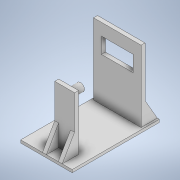
# Autodesk Inventor part: Część2
Saved by Autodesk Inventor 2022.2 (Build 262287010, 287A)
## iProperties
Created: 2023-01-23
Part Number: Część2
Material: Ogólny
Document SubType Name: Modeling
Designer: Miki
Density: 1 g/cm^3
Appearance: Domyślna
Author: Miki
Autodesk Inventor part; units mm, degrees
ref_plane "YZ Plane" through (0, 0, 0) normal (1, 0, 0) x (0, 1, 0)
ref_plane "XZ Plane" through (0, 0, 0) normal (0, 1, 0) x (-1, 0, 0)
ref_plane "XY Plane" through (0, 0, 0) normal (0, 0, 1) x (1, 0, 0)
sketch "Szkic1" plane through (0, 0, 0) normal (0, 1, 0) x (-1, 0, 0)
  line L0 (-25, 55) -> (40, 55)
  line L1 (40, 55) -> (40, -55)
  line L2 (40, -55) -> (-25, -55)
  line L3 (-25, -55) -> (-25, 55)
  point P0 (0, 0)
  point P1 (-25, 0)
  point P2 (40, 0)
  dimension "d0" = 65
  dimension "d1" = 110
  dimension "d2" = 55
  dimension "d25" = 40
  constraints: 8 end point, 2 midpoint, 2 parallel, 1 horizontal, 1 perpendicular
  measures "d0" distance of L1.end L2.end
  measures "d1" distance of L0.end L1.end
  measures "d2" vertical distance of point (0, 0) L2.end
  measures "d25" distance of point (0, 0) point (40, 0)
extrude "Wyciągnięcie proste1" add sketch "Szkic1" along normal blind 3.5
sketch "Szkic2" plane through (0, 3.5, 0) normal (0, 1, 0) x (1, 0, 0)
  line L0 (12.5, -39.5) -> (-12.5, -39.5)
  line L1 (-12.5, -39.5) -> (-12.5, -34.5)
  line L2 (-12.5, -34.5) -> (12.5, -34.5)
  line L3 (12.5, -34.5) -> (12.5, -39.5)
  point P0 (0, 0)
  point P1 (0, -34.5)
  dimension "d6" = 25
  dimension "d7" = 5
  dimension "d8" = 34.5
  dimension "d9" = 12.5
  constraints: 8 end point, 2 parallel, 1 horizontal, 1 midpoint, 1 perpendicular
  measures "d6" distance of L1.end L2.end
  measures "d7" distance of L0.end L1.end
  measures "d8" distance of point (0, 0) point (0, -34.5)
  measures "d9" horizontal distance of point (0, 0) L1.end
extrude "Wyciągnięcie proste2" add sketch "Szkic2" along normal blind 70
sketch "Szkic3" plane through (12.5, 3.5, 34.5) normal (0, 0, -1) x (-1, 0, 0)
  circle A0 centre (12.5, 60) radius 4.5
  line L0 (-12.5, 0) -> (52.5, 0) projected
  line L1 (25, 0) -> (25, 70) projected
  point P0 (12.5, -3.5)
  dimension "d16" = 9
  dimension "d17" = 60
  dimension "d18" = 12.5
  constraints: 1 centre point
  measures "d16" diameter of A0
  measures "d17" distance from line of L0 A0.centre
  measures "d18" distance from line of L1 A0.centre
extrude "Wyciągnięcie proste3" cut sketch "Szkic3" against normal up to next
sketch "Szkic4" plane through (0, 3.5, 0) normal (0, 1, 0) x (1, 0, 0)
  line L0 (-32.5, 34.5) -> (17.5, 34.5)
  line L1 (17.5, 34.5) -> (17.5, 39.5)
  line L2 (17.5, 39.5) -> (-32.5, 39.5)
  line L3 (-32.5, 39.5) -> (-32.5, 34.5)
  line L4 (12.5, -34.5) -> (-12.5, -34.5) projected
  line L5 (25, -55) -> (25, 55) projected
  point P0 (0, 0)
  point P1 (-7.5, 39.5)
  point P2 (17.5, 37)
  dimension "d22" = 50
  dimension "d23" = 5
  dimension "d24" = 69
  dimension "d26" = 7.5
  constraints: 8 end point, 2 midpoint, 2 parallel, 1 perpendicular
  measures "d22" distance of L2.end L1.end
  measures "d23" distance of L1.end L0.end
  measures "d24" distance between parallel lines of L0 L4
  measures "d26" distance from line of L5 point (17.5, 37)
extrude "Wyciągnięcie proste4" add sketch "Szkic4" along normal blind 90
sketch "Szkic5" plane through (17.5, 3.5, -39.5) normal (0, 0, -1) x (-1, 0, 0)
  line L0 (5, 75) -> (45, 75)
  line L1 (45, 75) -> (45, 55)
  line L2 (45, 55) -> (5, 55)
  line L3 (5, 55) -> (5, 75)
  line L4 (0, 0) -> (0, 90) projected
  line L5 (-7.5, 0) -> (57.5, 0) projected
  point P0 (17.5, -3.5)
  point P1 (45, 65)
  dimension "d29" = 40
  dimension "d30" = 20
  dimension "d31" = 5
  dimension "d33" = 65
  constraints: 8 end point, 2 parallel, 1 horizontal, 1 midpoint, 1 perpendicular
  measures "d29" distance of L1.end L2.end
  measures "d30" distance of L0.end L1.end
  measures "d31" distance between parallel lines of L4 L3
  measures "d33" distance from line of L5 point (45, 65)
extrude "Wyciągnięcie proste5" cut sketch "Szkic5" against normal up to next
sketch "Szkic6" plane through (-32.5, 3.5, -39.5) normal (-1, 0, 0) x (0, 0, 1)
  line L0 (-15.5, 0) -> (94.5, 0) projected
  line L1 (-15.5, 0) -> (0, 26.8468)
  line L2 (-15.5, 0) -> (15.5, 0) construction
  line L3 (0, 0) -> (0, 90) projected
  line L4 (0, 26.8468) -> (0, 0)
  line L5 (0, 0) -> (-15.5, 0)
  point P0 (39.5, -3.5)
  dimension "d36" = 60
  constraints: 8 end point, 1 collinear, 1 equal length, 1 horizontal, 1 perpendicular, 1 point on line, 1 vertical alignment
  measures "d36" angle of L2 L1
extrude "Wyciągnięcie proste6" add sketch "Szkic6" along normal mid plane 10
sketch "Szkic7" plane through (17.5, 3.5, -34.5) normal (1, 0, 0) x (0, 0, -1)
  line L0 (0, 0) -> (5, 0) projected
  line L1 (5, 26.8468) -> (20.5, 0) projected
  line L2 (20.5, 0) -> (5, 26.8468)
  line L3 (5, 26.8468) -> (5, 0)
  line L4 (5, 0) -> (20.5, 0)
  point P0 (-34.5, -3.5)
  point P1 (5, 0)
  constraints: 6 end point, 1 collinear, 1 perpendicular, 1 vertical
extrude "Wyciągnięcie proste7" add sketch "Szkic7" along normal mid plane 10
sketch "Szkic8" plane through (12.5, 3.5, 39.5) normal (1, 0, 0) x (0, 0, -1)
  line L0 (-15.5, 0) -> (94.5, 0) projected
  line L1 (-15.5, 0) -> (0, 26.8468)
  line L2 (-15.5, 0) -> (15.5, 0) construction
  line L3 (0, 0) -> (0, 70) projected
  line L4 (0, 26.8468) -> (0, 0)
  line L5 (0, 0) -> (-15.5, 0)
  point P0 (39.5, -3.5)
  dimension "d41" = 60
  constraints: 8 end point, 2 collinear, 1 equal length, 1 horizontal, 1 vertical alignment
  measures "d41" angle of L2 L1
extrude "Wyciągnięcie proste8" add sketch "Szkic8" against normal blind 5
sketch "Szkic9" plane through (-12.5, 3.5, 34.5) normal (-1, 0, 0) x (0, 0, 1)
  line L0 (-89.5, 0) -> (20.5, 0) projected
  line L1 (20.5, 0) -> (5, 26.8468)
  line L2 (5, 0) -> (5, 70) projected
  line L3 (20.5, -3.5) -> (20.5, 0) projected
  line L4 (5, 0) -> (20.5, 0)
  line L5 (5, 0) -> (0, 0) projected
  line L6 (5, 26.8468) -> (5, 0)
  line L7 (5, 0) -> (20.5, 0)
  point P0 (-34.5, -3.5)
  dimension "d44" = 120
  constraints: 8 end point, 1 horizontal, 1 perpendicular, 1 point on line, 1 vertical
  measures "d44" angle of L0 L1
extrude "Wyciągnięcie proste9" add sketch "Szkic9" against normal blind 5
sketch "Szkic10" plane through (0, 3.5, 0) normal (0, 1, 0) x (1, 0, 0)
  line L0 (17.5, 34.5) -> (17.5, 39.5) projected
  line L1 (17.5, 34.5) -> (22.5, 34.5)
  line L2 (22.5, 34.5) -> (22.5, 39.5)
  line L3 (22.5, 39.5) -> (17.5, 39.5)
  line L4 (17.5, 39.5) -> (17.5, 34.5)
  line L5 (-32.5, 39.5) -> (-32.5, 34.5) projected
  line L6 (-32.5, 34.5) -> (-37.5, 34.5)
  line L7 (-37.5, 34.5) -> (-37.5, 39.5)
  line L8 (-37.5, 39.5) -> (-32.5, 39.5)
  line L9 (-32.5, 39.5) -> (-32.5, 34.5)
  point P0 (0, 0)
  dimension "d47" = 5
  dimension "d48" = 5
  dimension "d49" = 5
  constraints: 16 end point, 4 parallel, 2 horizontal, 2 perpendicular, 1 point on line
  measures "d47" distance of L3.end L2.end
  measures "d48" distance of L2.end L1.end
  measures "d49" distance of L7.end L8.end
extrude "Wyciągnięcie proste10" add sketch "Szkic10" along normal blind 90
sketch "Szkic11" plane through (12.5, 3.5, 34.5) normal (0, 0, -1) x (-1, 0, 0)
  circle A0 centre (12.5, 60) radius 4.5 projected
  circle A1 centre (12.5, 60) radius 4.5
  line L0 (0, 55) -> (0, 75) projected
  point P0 (12.5, -3.5)
  constraints: 1 centre point, 1 coincident
extrude "Wyciągnięcie proste11" add sketch "Szkic11" against normal blind 5
sketch "Szkic12" plane through (12.5, 3.5, 34.5) normal (0, 0, -1) x (-1, 0, 0)
  circle A0 centre (12.5, 60) radius 5
  line L0 (0, 70) -> (25, 70) projected
  line L1 (25, 0) -> (25, 70) projected
  point P0 (12.5, -3.5)
  dimension "d55" = 10
  dimension "d56" = 10
  dimension "d57" = 12.5
  constraints: 1 centre point
  measures "d55" diameter of A0
  measures "d56" distance from line of L0 A0.centre
  measures "d57" distance from line of L1 A0.centre
extrude "Wyciągnięcie proste12" add sketch "Szkic12" along normal blind 15
